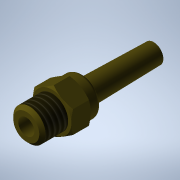
# Autodesk Inventor part: 1205858 AMTE-M-LH-M5
Saved by Autodesk Inventor 2021 (Build 250183000, 183)
## iProperties
Created: 2026-04-10
Part Number: 1205858 AMTE-M-LH-M5
Material: Generic
Catalog Web Link: www.3dfindit.com
Description: AMTE-silencer
Vendor: FESTO
Document SubType Name: Modeling
Designer: psAdmin
Manufacturer: FESTO
Mass: 1.5 g
Surface Area: 3.48765 cm^2
Volume: 0.285948 cm^3
Density: 1 g/cm^3
Appearance: PSOLRGB-209-199-99
Category: PARTsolutions
Company: FESTO
Title: 1205858 AMTE-M-LH-M5
Author: Cadenas PARTsolutions
Comments: silencer
PSOL_IDENT_0: {$CADENAS_DATA/23d-libs/festo/parts/a/amte/amte.prj},178 {VTYP=3D},{NB=1205858 AMTE-M-LH-M5},{LINA=1
PSOL_IDENT_1: 205858 AMTE-M-LH-M5},{NN=AMTE},{DATE=25.06.2025 12:56:18},{GEOMDATE=23.06.2025 13:31:03},{VERSION=},
PSOL_IDENT_2: {LINEID=20},{WBVAR=},{WBNUMERIC=}  {NB=1205858 AMTE-M-LH-M5},{LINA=1205858 AMTE-M-LH-M5},{KT=DUMMY},
PSOL_IDENT_3: {TNR=1205858},{TYP=AMTE-M-LH-M5},{D1=M5},{ZOLL=-},{D2=3.0},{D3=2.50},{L1=19.8},{L2=4.0},{L3=3.0},{SW=
PSOL_IDENT_4: 6.0},{SW1=0.000},{VERS=1},{A1=5.000},{B2=1.700},{D4=3.483},{D5=5.800},{R=0.500},{CNSMASSEXACT=0.0015
PSOL_IDENT_5: },{GTIN=4052568061586},{REACH=Ja},{REACHSVHC=Ja},{REACHHAZSUBS=7439-92-1},{REACHSCIP=099e2c8b-2252-4
PSOL_IDENT_6: 414-bb57-4036a0cc366b},{REACHVALDATE=05.03.2025}
NB: 1205858 AMTE-M-LH-M5
NN: AMTE
NT: silencer
NBSYN: $TNR. $TYP.
LINA: 1205858 AMTE-M-LH-M5
CATALOG: Festo
TNR: 1205858
TYP: AMTE-M-LH-M5
D1: M5
D2: 3
D3: 2.5
L1: 19.8
L2: 4
L3: 3
SW: 6
SW1: 0
CNSMASSEXACT: 0.0015
GTIN: 4052568061586
REACH: Yes
REACHSVHC: Yes
REACHHAZSUBS: 7439-92-1
REACHVALDATE: 05.03.2025
SUPPLIER: FESTO
ARTICLENO: 1205858 AMTE-M-LH-M5
BOMINFO: 1205858 AMTE-M-LH-M5
CREATOR: CADENAS GmbH
Autodesk Inventor part; units mm, degrees
sketch "Sketch_1" plane through (0, 0, 0) normal (1, 0, 0) x (0, 1, 0)
  line L0 (0, -19.8) -> (0, 0)
  line L1 (0, -4) -> (1.25, -4)
  line L2 (1.25, -4) -> (1.25, 0)
  line L3 (1.25, 0) -> (2.0095, 0)
  line L4 (2.0095, 0) -> (2.5, -0.4905)
  line L5 (2.5, -0.4905) -> (2.5, -4)
  line L6 (2.5, -4) -> (3, -4)
  line L7 (3, -4) -> (3.6, -4.3464)
  line L8 (3.6, -4.3464) -> (3.6, -6.6536)
  line L9 (3.6, -6.6536) -> (3, -7)
  line L10 (3, -7) -> (2.9, -7)
  line L11 (2.9, -7) -> (2.9, -8.2)
  arc A0 (2.4, -8.7) -> (2.9, -8.2) centre (2.4, -8.2) ccw
  line L12 (2.4, -8.7) -> (1.7415, -8.7)
  line L13 (1.7415, -8.7) -> (1.5, -19.8)
  line L14 (1.5, -19.8) -> (0, -19.8)
  line L15 (0, -19.8) -> (0, -4)
  constraints: 32 end point, 2 point on circle, 1 centre point
revolve "Revolution1" add sketch "Sketch_1" angle 360 about axis through (0, 0, -19.8) along (0, 0, -1)
thread "Thread1" size "M5x0.8" class "6g" standard "ISO Metric profile" full length
sketch "Sketch_2" plane through (0, 0, -4) normal (0, 0, 1) x (1, 0, 0)
  line L0 (-6, 6) -> (-6, -6)
  line L1 (-6, -6) -> (6, -6)
  line L2 (6, -6) -> (6, 6)
  line L3 (6, 6) -> (-6, 6)
  line L4 (-3, -1.7321) -> (0, -3.4641)
  line L5 (0, -3.4641) -> (3, -1.7321)
  line L6 (3, -1.7321) -> (3, 1.7321)
  line L7 (3, 1.7321) -> (0, 3.4641)
  line L8 (0, 3.4641) -> (-3, 1.7321)
  line L9 (-3, 1.7321) -> (-3, -1.7321)
  constraints: 20 end point
extrude "Extrusion1" cut sketch "Sketch_2" against normal blind 3
ref_plane "ANBAU_XY" through (0, 0, -4) normal (0, 0, 1) x (1, 0, 0)
ref_plane "ANBAU_YZ" through (0, 0, -4) normal (1, 0, 0) x (0, 1, 0)
ref_plane "ANBAU_ZX" through (0, 0, -4) normal (0, 1, 0) x (0, 0, 1)
ref_plane "ANBAU_STD_XY" through (0, 0, -4) normal (0, 0, -1) x (1, 0, 0)
ref_plane "ANBAU_STD_YZ" through (0, 0, -4) normal (1, 0, 0) x (0, -1, 0)
ref_plane "ANBAU_STD_ZX" through (0, 0, -4) normal (0, -1, 0) x (0, 0, -1)
body "Solid1"
